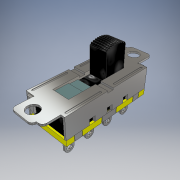
# Autodesk Inventor part: Switch-46300LDRX
Saved by Autodesk Inventor 2018 (Build 220112000, 112)
## iProperties
Created: 2021-02-17
Part Number: Switch-46300LDRX
Material: Všeobecné
Document SubType Name: Modeling
Designer: Jozko Mrkvicka
Density: 1 g/cm^3
Appearance: Výchozí
Author: Jozko Mrkvicka
Autodesk Inventor part; units mm, degrees
ref_plane "YZ Plane" through (0, 0, 0) normal (1, 0, 0) x (0, 1, 0)
ref_plane "XZ Plane" through (0, 0, 0) normal (0, 1, 0) x (-1, 0, 0)
sketch "Náčrt1" plane through (0, 0, 0) normal (0, 1, 0) x (-1, 0, 0)
  line L0 (-2.54, 20.955) -> (2.54, 20.955)
  line L1 (2.54, -20.955) -> (-2.54, -20.955)
  line L2 (-3.81, -19.685) -> (-3.81, -15.24)
  line L3 (3.81, 19.685) -> (3.81, 15.24)
  line L4 (5.715, -14.605) -> (5.715, -18.415)
  line L5 (4.445, -19.685) -> (3.81, -19.685)
  line L6 (-5.715, 14.605) -> (-5.715, 18.415)
  line L7 (-4.445, 19.685) -> (-3.81, 19.685)
  circle A0 centre (0, -17.78) radius 1.905
  circle A1 centre (0, 17.78) radius 1.905
  line L8 (-2.8575, 9.8425) -> (2.8575, 9.8425)
  line L9 (2.8575, -9.8425) -> (-2.8575, -9.8425)
  line L10 (6.985, -14.605) -> (5.715, -14.605)
  line L11 (-5.715, -14.605) -> (-6.985, -14.605)
  line L12 (6.985, 14.605) -> (6.985, 0.9525)
  line L13 (6.985, -0.9525) -> (6.985, -14.605)
  line L14 (3.81, 19.685) -> (3.81, 15.24)
  line L15 (3.81, -19.685) -> (3.81, -19.685)
  line L16 (2.8575, 9.8425) -> (2.8575, 0.9525)
  line L17 (2.8575, -0.9525) -> (2.8575, -9.8425)
  line L18 (-6.985, 0.9525) -> (-2.8575, 0.9525)
  line L19 (2.8575, 0.9525) -> (6.985, 0.9525)
  line L20 (6.985, -0.9525) -> (2.8575, -0.9525)
  line L21 (-2.8575, -0.9525) -> (-6.985, -0.9525)
  line L22 (-2.8575, -9.8425) -> (-2.8575, -0.9525)
  line L23 (-2.8575, 0.9525) -> (-2.8575, 9.8425)
  line L24 (-3.81, -20.955) -> (-3.81, -15.24)
  line L25 (-3.81, 19.685) -> (-3.81, 19.685)
  line L26 (-6.985, -14.605) -> (-6.985, -0.9525)
  line L27 (-6.985, 0.9525) -> (-6.985, 14.605)
  line L28 (6.985, 14.605) -> (5.715, 14.605)
  line L29 (-5.715, 14.605) -> (-6.985, 14.605)
  arc A2 (3.81, 19.685) -> (2.54, 20.955) centre (2.54, 19.685) ccw
  arc A3 (-2.54, 20.955) -> (-3.81, 19.685) centre (-2.54, 19.685) ccw
  arc A4 (-4.445, 19.685) -> (-5.715, 18.415) centre (-4.445, 18.415) ccw
  arc A5 (4.445, -19.685) -> (5.715, -18.415) centre (4.445, -18.415) ccw
  arc A6 (-3.81, -19.685) -> (-2.54, -20.955) centre (-2.54, -19.685) ccw
  arc A7 (2.54, -20.955) -> (3.81, -19.685) centre (2.54, -19.685) ccw
  line L30 (-5.715, -14.605) -> (-5.715, -15.24)
  line L31 (-5.715, -15.24) -> (-3.81, -15.24)
  line L32 (5.715, 14.605) -> (5.715, 15.24)
  line L33 (5.715, 15.24) -> (3.81, 15.24)
  point P0 (0, 0)
  dimension "d14" = 1.27
  dimension "d15" = 1.27
  constraints: 68 end point, 18 parallel, 12 point on circle, 12 tangent, 8 centre point, 6 horizontal, 4 equal radius, 4 perpendicular, 2 point on line, 4 other
  measures "d14" radius of A2
  measures "d15" radius of A3
extrude "Vysunutí1" add sketch "Náčrt1" along normal blind 0.635
sketch "Náčrt2" plane through (0, 0, 0) normal (0, -1, 0) x (1, 0, 0)
  line L0 (5.715, 14.605) -> (6.985, 14.605) projected
  line L1 (-6.985, -0.9525) -> (-6.985, -14.605) projected
  line L2 (6.985, 14.605) -> (-6.985, 14.605)
  line L3 (-6.985, 14.605) -> (-6.985, -14.605)
  line L4 (-6.985, -14.605) -> (6.985, -14.605)
  line L5 (6.985, -14.605) -> (6.985, 14.605)
  constraints: 8 end point, 2 parallel, 1 horizontal, 1 perpendicular
extrude "Vysunutí2" add sketch "Náčrt2" along normal blind 6.35
sketch "Náčrt3" plane through (0, 0.635, 0) normal (0, 1, 0) x (1, 0, 0)
  line L0 (-5.715, -2.54) -> (-5.715, -13.335)
  line L1 (-6.35, -13.335) -> (-6.35, -2.54)
  arc A0 (-6.35, -13.335) -> (-5.715, -13.335) centre (-6.0325, -13.335) ccw
  arc A1 (-5.715, -2.54) -> (-6.35, -2.54) centre (-6.0325, -2.54) ccw
  line L2 (-5.715, 2.54) -> (-5.715, 13.335)
  line L3 (-6.35, 13.335) -> (-6.35, 2.54)
  arc A2 (-5.715, 13.335) -> (-6.35, 13.335) centre (-6.0325, 13.335) ccw
  arc A3 (-6.35, 2.54) -> (-5.715, 2.54) centre (-6.0325, 2.54) ccw
  line L4 (5.715, -2.54) -> (5.715, -13.335)
  line L5 (6.35, -13.335) -> (6.35, -2.54)
  arc A4 (5.715, -13.335) -> (6.35, -13.335) centre (6.0325, -13.335) ccw
  arc A5 (6.35, -2.54) -> (5.715, -2.54) centre (6.0325, -2.54) ccw
  line L6 (5.715, 2.54) -> (5.715, 13.335)
  line L7 (6.35, 13.335) -> (6.35, 2.54)
  arc A6 (6.35, 13.335) -> (5.715, 13.335) centre (6.0325, 13.335) ccw
  arc A7 (5.715, 2.54) -> (6.35, 2.54) centre (6.0325, 2.54) ccw
  point P0 (-6.985, -0.9525)
  constraints: 16 end point, 16 point on circle, 8 centre point, 1 parallel
extrude "Vysunutí3" cut sketch "Náčrt3" against normal blind 0.1588
sketch "Náčrt4" plane through (0, 0, 0) normal (0, 1, 0) x (1, 0, 0)
  line L0 (2.8575, -0.9525) -> (2.8575, -9.8425) projected
  line L1 (-2.8575, -9.8425) -> (2.8575, -9.8425)
  line L2 (2.8575, -9.8425) -> (2.8575, -2.8575)
  line L3 (2.8575, -2.8575) -> (-2.8575, -2.8575)
  line L4 (-2.8575, -2.8575) -> (-2.8575, -9.8425)
  point P0 (0, 0)
  dimension "d30" = 6.985
  constraints: 8 end point, 2 parallel, 1 horizontal, 1 perpendicular, 1 point on line
  measures "d30" distance of L2.end L1.end
extrude "Vysunutí4" add sketch "Náčrt4" along normal blind 8.89
sketch "Náčrt5" plane through (2.8575, 0.635, 2.8575) normal (1, 0, 0) x (0, 0, -1)
  arc A0 (0, 7.3576) -> (-6.985, 7.3576) centre (-3.4925, 1.0099) ccw
  line L0 (0, 8.7121) -> (-6.985, 8.7121)
  line L1 (-6.985, 7.3576) -> (-6.985, 8.7121)
  line L2 (0, 7.3576) -> (0, 8.7121)
  constraints: 6 end point, 2 point on circle, 1 centre point
extrude "Vysunutí5" cut sketch "Náčrt5" against normal up to next
sketch "Náčrt6" plane through (2.8575, 0.635, 9.8425) normal (1, 0, 0) x (0, 0, -1)
  circle A0 centre (0.5108, 7.613) radius 0.3175
  circle A1 centre (1.2173, 7.8885) radius 0.3175
  circle A2 centre (1.9488, 8.0886) radius 0.3175
  circle A3 centre (2.6971, 8.2112) radius 0.3175
  circle A4 centre (3.4542, 8.2549) radius 0.3175
  circle A5 centre (4.2118, 8.2192) radius 0.3175
  circle A6 centre (4.9614, 8.1045) radius 0.3175
  circle A7 centre (5.6949, 7.9121) radius 0.3175
  circle A8 centre (6.4043, 7.6441) radius 0.3175
  point P0 (3.4925, 1.0099)
  point P1 (9.8425, -0.635)
  point P2 (3.4925, 1.0099)
  point P3 (3.4925, 1.0099)
  point P4 (3.4925, 1.0099)
  point P5 (3.4925, 1.0099)
  point P6 (3.4925, 1.0099)
  point P7 (3.4925, 1.0099)
  point P8 (3.4925, 1.0099)
  point P9 (3.4925, 1.0099)
  dimension "d38" = 48
  constraints: 9 centre point, 1 coincident, 24 other
extrude "Vysunutí6" add sketch "Náčrt6" against normal up to surface (5.715 mm away)
sketch "Náčrt7" plane through (0, 0, 0) normal (0, 1, 0) x (1, 0, 0)
  line L0 (2.8575, 0.9525) -> (2.8575, 9.8425) projected
  line L1 (-2.8575, -2.8575) -> (2.8575, -2.8575)
  line L2 (2.8575, -2.8575) -> (2.8575, 4.7625)
  line L3 (2.8575, 4.7625) -> (-2.8575, 4.7625)
  line L4 (-2.8575, 4.7625) -> (-2.8575, -2.8575)
  point P0 (0, 0)
  dimension "d42" = 7.62
  constraints: 8 end point, 2 parallel, 1 horizontal, 1 perpendicular, 1 point on line
  measures "d42" distance of L2.end L1.end
extrude "Vysunutí7" cut sketch "Náčrt7" against normal blind 0.3175
sketch "Náčrt8" plane through (0, -0.3175, 0) normal (0, 1, 0) x (1, 0, 0)
  line L0 (2.8575, -2.8575) -> (-2.8575, -2.8575) projected
  line L1 (2.8575, 4.7625) -> (2.8575, -2.8575) projected
  line L2 (-2.8575, -2.8575) -> (2.8575, -2.8575)
  line L3 (2.8575, -2.8575) -> (2.8575, 1.5875)
  line L4 (2.8575, 1.5875) -> (-2.8575, 1.5875)
  line L5 (-2.8575, 1.5875) -> (-2.8575, -2.8575)
  point P0 (0, 0)
  dimension "d45" = 4.445
  constraints: 8 end point, 2 parallel, 1 horizontal, 1 perpendicular, 1 point on line
  measures "d45" distance of L3.end L2.end
extrude "Vysunutí8" cut sketch "Náčrt8" against normal blind 0.3175
sketch "Náčrt9" plane through (0, -6.35, 0) normal (0, -1, 0) x (1, 0, 0)
  line L0 (6.35, 2.8575) -> (6.985, 2.8575)
  line L1 (6.985, -2.8575) -> (6.35, -2.8575)
  line L2 (6.35, -2.8575) -> (6.35, 2.8575)
  line L3 (-6.985, 2.8575) -> (-6.35, 2.8575)
  line L4 (-6.35, 2.8575) -> (-6.35, -2.8575)
  line L5 (-6.35, -2.8575) -> (-6.985, -2.8575)
  line L6 (6.35, 12.065) -> (6.35, 9.525)
  line L7 (6.35, 9.525) -> (6.985, 9.525)
  line L8 (6.985, 12.065) -> (6.35, 12.065)
  line L9 (-6.985, 12.065) -> (-6.35, 12.065)
  line L10 (-6.35, 12.065) -> (-6.35, 9.525)
  line L11 (-6.35, 9.525) -> (-6.985, 9.525)
  line L12 (6.985, -12.065) -> (6.35, -12.065)
  line L13 (6.35, -12.065) -> (6.35, -9.525)
  line L14 (6.35, -9.525) -> (6.985, -9.525)
  line L15 (-6.985, -12.065) -> (-6.35, -12.065)
  line L16 (-6.35, -12.065) -> (-6.35, -9.525)
  line L17 (-6.35, -9.525) -> (-6.985, -9.525)
  line L18 (6.985, 14.605) -> (-6.985, 14.605) projected
  line L19 (6.985, 14.605) -> (-6.985, 14.605)
  line L20 (-6.985, -14.605) -> (6.985, -14.605)
  line L21 (6.985, 12.065) -> (6.985, 14.605)
  line L22 (6.985, 2.8575) -> (6.985, 9.525)
  line L23 (6.985, -14.605) -> (6.985, -12.065)
  line L24 (6.985, -9.525) -> (6.985, -2.8575)
  line L25 (-6.985, -12.065) -> (-6.985, -14.605)
  line L26 (-6.985, -2.8575) -> (-6.985, -9.525)
  line L27 (-6.985, 14.605) -> (-6.985, 12.065)
  line L28 (-6.985, 9.525) -> (-6.985, 2.8575)
  point P0 (0, 0)
  point P1 (6.985, 0)
  point P2 (-6.985, 0)
  constraints: 56 end point, 22 parallel, 8 perpendicular, 6 horizontal, 3 point on line
extrude "Vysunutí9" add sketch "Náčrt9" along normal blind 1.905
sketch "Náčrt10" plane through (0, -6.35, 0) normal (0, -1, 0) x (1, 0, 0)
  line L0 (-6.985, -11.938) -> (-6.477, -11.938)
  line L1 (-6.477, -11.938) -> (-6.477, -9.652)
  line L2 (-6.477, -9.652) -> (-6.985, -9.652)
  line L3 (-6.477, 9.652) -> (-6.985, 9.652)
  line L4 (-6.985, 11.938) -> (-6.477, 11.938)
  line L5 (-6.477, 11.938) -> (-6.477, 9.652)
  line L6 (6.477, 9.652) -> (6.985, 9.652)
  line L7 (6.985, 11.938) -> (6.477, 11.938)
  line L8 (6.477, 11.938) -> (6.477, 9.652)
  line L9 (6.477, -11.938) -> (6.985, -11.938)
  line L10 (6.985, -9.652) -> (6.477, -9.652)
  line L11 (6.477, -9.652) -> (6.477, -11.938)
  line L12 (-6.477, -2.54) -> (-6.985, -2.54)
  line L13 (-6.985, 2.54) -> (-6.477, 2.54)
  line L14 (-6.477, 2.54) -> (-6.477, -2.54)
  line L15 (6.477, -2.54) -> (6.985, -2.54)
  line L16 (6.985, 2.54) -> (6.477, 2.54)
  line L17 (6.477, 2.54) -> (6.477, -2.54)
  line L18 (-6.985, -11.938) -> (-6.985, -9.652)
  line L19 (-6.985, -2.54) -> (-6.985, 2.54)
  line L20 (-6.985, 9.652) -> (-6.985, 11.938)
  line L21 (6.985, 9.652) -> (6.985, 11.938)
  line L22 (6.985, -2.54) -> (6.985, 2.54)
  line L23 (6.985, -11.938) -> (6.985, -9.652)
  point P0 (0, 0)
  point P1 (-6.985, -10.795)
  point P2 (-6.985, 10.795)
  point P3 (6.985, 10.795)
  point P4 (6.985, -10.795)
  point P5 (-6.985, 0)
  point P6 (6.985, 0)
  constraints: 48 end point, 6 horizontal, 6 parallel, 1 perpendicular
extrude "Vysunutí10" add sketch "Náčrt10" along normal blind 1.905
ref_plane "Pracovní rovina1" through (-6.477, -6.35, -2.54) normal (0, -1, 0) x (1, 0, 0)
split_face "Rozdělit1"
sketch "Náčrt11" plane through (0, -8.255, 0) normal (0, -1, 0) x (1, 0, 0)
  line L0 (-6.985, -12.065) -> (-6.985, -14.605) projected
  line L1 (-3.4925, -12.3896) -> (-3.4925, -9.2087)
  line L2 (-2.8575, -9.2087) -> (-2.8575, -12.3896)
  arc A0 (-3.4925, -9.2087) -> (-4.3905, -8.3107) centre (-4.5023, -9.3205) ccw
  arc A1 (-2.8575, -9.2087) -> (-4.0571, -7.7332) centre (-4.5023, -9.3205) ccw
  arc A2 (-2.8575, -12.3896) -> (-1.9595, -13.2876) centre (-1.8477, -12.2777) ccw
  arc A3 (-3.4925, -12.3896) -> (-2.3035, -13.8835) centre (-1.9595, -12.3896) ccw
  line L3 (-1.9595, -13.2876) -> (-2.3035, -13.8835)
  line L4 (-4.3905, -8.3107) -> (-4.0571, -7.7332)
  line L5 (-4.3905, -1.1733) -> (-4.0571, -0.5958)
  arc A4 (-2.8575, -2.0713) -> (-4.0571, -0.5958) centre (-4.5023, -2.1831) ccw
  arc A5 (-3.4925, -2.0713) -> (-4.3905, -1.1733) centre (-4.5023, -2.1831) ccw
  line L6 (-3.4925, -5.2522) -> (-3.4925, -2.0713)
  line L7 (-2.8575, -2.0713) -> (-2.8575, -5.2522)
  arc A6 (-2.8575, -5.2522) -> (-1.9595, -6.1502) centre (-1.8477, -5.1403) ccw
  arc A7 (-3.4925, -5.2522) -> (-2.3035, -6.7461) centre (-1.9595, -5.2522) ccw
  line L8 (-1.9595, -6.1502) -> (-2.3035, -6.7461)
  line L9 (-4.3905, 5.9641) -> (-4.0571, 6.5416)
  arc A8 (-2.8575, 5.0661) -> (-4.0571, 6.5416) centre (-4.5023, 4.9543) ccw
  arc A9 (-3.4925, 5.0661) -> (-4.3905, 5.9641) centre (-4.5023, 4.9543) ccw
  line L10 (-3.4925, 1.8852) -> (-3.4925, 5.0661)
  line L11 (-2.8575, 5.0661) -> (-2.8575, 1.8852)
  arc A10 (-2.8575, 1.8852) -> (-1.9595, 0.9872) centre (-1.8477, 1.9971) ccw
  arc A11 (-3.4925, 1.8852) -> (-2.3035, 0.3913) centre (-1.9595, 1.8852) ccw
  line L12 (-1.9595, 0.9872) -> (-2.3035, 0.3913)
  line L13 (-4.3905, 13.1015) -> (-4.0571, 13.679)
  arc A12 (-2.8575, 12.2035) -> (-4.0571, 13.679) centre (-4.5023, 12.0917) ccw
  arc A13 (-3.4925, 12.2035) -> (-4.3905, 13.1015) centre (-4.5023, 12.0917) ccw
  line L14 (-3.4925, 9.0226) -> (-3.4925, 12.2035)
  line L15 (-2.8575, 12.2035) -> (-2.8575, 9.0226)
  arc A14 (-2.8575, 9.0226) -> (-1.9595, 8.1246) centre (-1.8477, 9.1345) ccw
  arc A15 (-3.4925, 9.0226) -> (-2.3035, 7.5287) centre (-1.9595, 9.0226) ccw
  line L16 (-1.9595, 8.1246) -> (-2.3035, 7.5287)
  point P0 (-3.175, -10.7991)
  point P1 (-3.175, -3.6617)
  point P2 (-3.175, 3.4757)
  point P3 (-3.175, 10.6131)
  dimension "d84" = 7.1374
  constraints: 32 end point, 32 point on circle, 16 centre point, 4 concentric, 2 parallel, 1 tangent, 1 vertical, 64 other
  measures "d84" distance of L4.end L5.end
extrude "Vysunutí11" add sketch "Náčrt11" along normal blind 0.635
sketch "Náčrt12" plane through (0, -8.89, 0) normal (0, -1, 0) x (1, 0, 0)
  line L0 (-3.4925, -12.3896) -> (-3.4925, -9.2087) projected
  line L1 (-2.8575, -9.2087) -> (-2.8575, -12.3896) projected
  line L2 (-3.4925, -12.3866) -> (-2.8575, -12.3866)
  line L3 (-2.8575, -12.3866) -> (-2.8575, -9.2116)
  line L4 (-2.8575, -9.2116) -> (-3.4925, -9.2116)
  line L5 (-3.4925, -9.2116) -> (-3.4925, -12.3866)
  line L6 (-3.4925, -2.0742) -> (-3.4925, -5.2492)
  line L7 (-3.4925, -5.2492) -> (-2.8575, -5.2492)
  line L8 (-2.8575, -2.0742) -> (-3.4925, -2.0742)
  line L9 (-2.8575, -5.2492) -> (-2.8575, -2.0742)
  line L10 (-3.4925, 5.0632) -> (-3.4925, 1.8882)
  line L11 (-3.4925, 1.8882) -> (-2.8575, 1.8882)
  line L12 (-2.8575, 5.0632) -> (-3.4925, 5.0632)
  line L13 (-2.8575, 1.8882) -> (-2.8575, 5.0632)
  line L14 (-3.4925, 12.2006) -> (-3.4925, 9.0256)
  line L15 (-3.4925, 9.0256) -> (-2.8575, 9.0256)
  line L16 (-2.8575, 12.2006) -> (-3.4925, 12.2006)
  line L17 (-2.8575, 9.0256) -> (-2.8575, 12.2006)
  point P0 (0, 0)
  point P1 (-3.175, -10.7991)
  dimension "d91" = 3.175
  dimension "d94" = 7.1374
  constraints: 32 end point, 2 parallel, 1 collinear, 1 horizontal, 1 perpendicular, 1 point on line, 1 vertical, 23 other
  measures "d91" distance of L3.end L2.end
  measures "d94" distance of L4.end L6.start
extrude "Vysunutí12" add sketch "Náčrt12" along normal blind 6.35
sketch "Náčrt13" plane through (-3.4925, -8.255, -12.3896) normal (-1, 0, 0) x (0, 0, 1)
  line L0 (3.1779, -1.27) -> (3.1779, -3.81)
  line L1 (0, -3.81) -> (0, -1.27)
  line L2 (2.5415, -1.27) -> (2.5415, -3.81)
  line L3 (0.6365, -3.81) -> (0.6365, -1.27)
  arc A0 (0.0029, -5.3975) -> (3.1779, -5.3975) centre (1.5904, -5.3975) ccw
  circle A1 centre (1.5904, -5.3975) radius 0.9525
  line L4 (3.175, -1.27) -> (2.5415, -1.27)
  line L5 (0.6365, -1.27) -> (0, -1.27)
  line L6 (0, -1.27) -> (0.6365, -1.27)
  line L7 (2.5415, -1.27) -> (3.1779, -1.27)
  line L8 (3.1779, -3.81) -> (2.5415, -3.81)
  line L9 (0.6365, -3.81) -> (0, -3.81)
  line L10 (3.1779, -5.3975) -> (3.1779, -7.479)
  line L11 (3.1779, -7.479) -> (0.0029, -7.479)
  line L12 (0.0029, -7.479) -> (0.0029, -5.3975)
  circle A2 centre (8.7278, -5.3975) radius 0.9525
  arc A3 (7.1403, -5.3975) -> (10.3153, -5.3975) centre (8.7278, -5.3975) ccw
  line L13 (10.3153, -7.479) -> (7.1403, -7.479)
  line L14 (7.1403, -7.479) -> (7.1403, -5.3975)
  line L15 (10.3153, -5.3975) -> (10.3153, -7.479)
  line L16 (10.3153, -3.81) -> (9.6789, -3.81)
  line L17 (7.7739, -3.81) -> (7.1374, -3.81)
  line L18 (10.3124, -1.27) -> (9.6789, -1.27)
  line L19 (9.6789, -1.27) -> (10.3153, -1.27)
  line L20 (7.7739, -3.81) -> (7.7739, -1.27)
  line L21 (7.1374, -3.81) -> (7.1374, -1.27)
  line L22 (7.7739, -1.27) -> (7.1374, -1.27)
  line L23 (7.1374, -1.27) -> (7.7739, -1.27)
  line L24 (9.6789, -1.27) -> (9.6789, -3.81)
  line L25 (10.3153, -1.27) -> (10.3153, -3.81)
  circle A4 centre (15.8652, -5.3975) radius 0.9525
  arc A5 (14.2777, -5.3975) -> (17.4527, -5.3975) centre (15.8652, -5.3975) ccw
  line L26 (17.4527, -7.479) -> (14.2777, -7.479)
  line L27 (14.2777, -7.479) -> (14.2777, -5.3975)
  line L28 (17.4527, -5.3975) -> (17.4527, -7.479)
  line L29 (17.4527, -3.81) -> (16.8163, -3.81)
  line L30 (14.9113, -3.81) -> (14.2748, -3.81)
  line L31 (17.4498, -1.27) -> (16.8163, -1.27)
  line L32 (16.8163, -1.27) -> (17.4527, -1.27)
  line L33 (14.9113, -3.81) -> (14.9113, -1.27)
  line L34 (14.2748, -3.81) -> (14.2748, -1.27)
  line L35 (14.9113, -1.27) -> (14.2748, -1.27)
  line L36 (14.2748, -1.27) -> (14.9113, -1.27)
  line L37 (16.8163, -1.27) -> (16.8163, -3.81)
  line L38 (17.4527, -1.27) -> (17.4527, -3.81)
  circle A6 centre (23.0026, -5.3975) radius 0.9525
  arc A7 (21.4151, -5.3975) -> (24.5901, -5.3975) centre (23.0026, -5.3975) ccw
  line L39 (24.5901, -7.479) -> (21.4151, -7.479)
  line L40 (21.4151, -7.479) -> (21.4151, -5.3975)
  line L41 (24.5901, -5.3975) -> (24.5901, -7.479)
  line L42 (24.5901, -3.81) -> (23.9537, -3.81)
  line L43 (22.0487, -3.81) -> (21.4122, -3.81)
  line L44 (24.5872, -1.27) -> (23.9537, -1.27)
  line L45 (23.9537, -1.27) -> (24.5901, -1.27)
  line L46 (22.0487, -3.81) -> (22.0487, -1.27)
  line L47 (21.4122, -3.81) -> (21.4122, -1.27)
  line L48 (22.0487, -1.27) -> (21.4122, -1.27)
  line L49 (21.4122, -1.27) -> (22.0487, -1.27)
  line L50 (23.9537, -1.27) -> (23.9537, -3.81)
  line L51 (24.5901, -1.27) -> (24.5901, -3.81)
  point P0 (0, 0)
  point P1 (12.3896, 8.255)
  dimension "d109" = 7.1374
  constraints: 104 end point, 8 centre point, 8 point on circle, 7 parallel, 4 coincident, 3 horizontal, 2 perpendicular, 1 collinear, 89 other
  measures "d109" distance of L10.start L15.start
extrude "Vysunutí13" cut sketch "Náčrt13" against normal up to next
sketch "Náčrt14" plane through (6.985, -6.35, -14.605) normal (0, 0, -1) x (-1, 0, 0)
  line L0 (0, 6.985) -> (0.635, 6.985)
  line L1 (13.97, 6.985) -> (13.335, 6.985)
  line L2 (13.335, 6.35) -> (0.635, 6.35)
  line L3 (0.635, 6.35) -> (0.635, 0)
  line L4 (0.635, 0) -> (13.335, 0)
  line L5 (13.335, 0) -> (13.335, 6.35)
  point P0 (6.985, 6.35)
  constraints: 12 end point, 3 horizontal, 2 parallel, 1 perpendicular
extrude "Vysunutí14" cut sketch "Náčrt14" against normal blind 0.635
sketch "Náčrt15" plane through (-6.985, -6.35, 14.605) normal (0, 0, 1) x (1, 0, 0)
  line L0 (13.335, 6.35) -> (0.635, 6.35) projected
  line L1 (13.335, 0) -> (13.335, 6.35) projected
  line L2 (0.635, 0) -> (13.335, 0) projected
  line L3 (0.635, 6.35) -> (0.635, 0) projected
  point P0 (6.985, 6.35)
extrude "Vysunutí15" cut sketch "Náčrt15" against normal blind 0.635
sketch "Náčrt16" plane through (0, 0, 0) normal (0, -1, 0) x (1, 0, 0)
  line L0 (-5.715, 15.24) -> (-3.81, 15.24)
  line L1 (-3.81, 15.24) -> (-3.81, 14.605)
  line L2 (-3.81, 14.605) -> (-5.715, 14.605)
  line L3 (-5.715, 14.605) -> (-5.715, 15.24)
  line L4 (5.715, -15.24) -> (3.81, -15.24) projected
  line L5 (5.715, -15.24) -> (3.81, -15.24)
  line L6 (3.81, -15.24) -> (3.81, -14.605)
  line L7 (3.81, -14.605) -> (5.715, -14.605)
  line L8 (5.715, -14.605) -> (5.715, -15.24)
  point P0 (0, 0)
  dimension "d120" = 1.905
  dimension "d121" = 0.635
  constraints: 16 end point, 4 parallel, 2 horizontal, 2 perpendicular
  measures "d120" distance of L6.end L7.end
  measures "d121" distance of L5.end L6.end
extrude "Vysunutí16" add sketch "Náčrt16" along normal blind 4.445
fillet "Zaoblení1" radius 1.905 2 edges at (5.715, -4.445, -14.9225) (-5.715, -4.445, 14.9225)
fillet "Zaoblení2" radius 0.635 2 edges at (-4.7625, 0.635, 15.24) (4.7625, 0.635, -15.24)
fillet "Zaoblení3" radius 0.3175 2 edges at (-4.7625, 0, 14.605) (4.7625, 0, -14.605)
sketch "Náčrt18" plane through (6.985, 0, 0.9525) normal (1, 0, 0) x (0, 0, -1)
  line L0 (-8.5725, -6.35) -> (-1.905, -6.35) projected
  line L1 (-1.5875, -6.35) -> (3.4925, -6.35) projected
  line L2 (3.81, -6.35) -> (10.4775, -6.35) projected
  line L3 (0, -6.35) -> (0, -4.445)
  line L4 (0, -4.445) -> (1.905, -4.445)
  line L5 (1.905, -4.445) -> (1.905, -6.35)
  line L6 (6.1912, -6.35) -> (6.1912, -4.445)
  line L7 (6.1912, -4.445) -> (8.0963, -4.445)
  line L8 (8.0963, -4.445) -> (8.0963, -6.35)
  line L9 (-4.2863, -6.35) -> (-4.2863, -4.445)
  line L10 (-4.2863, -4.445) -> (-6.1913, -4.445)
  line L11 (-6.1913, -4.445) -> (-6.1913, -6.35)
  line L12 (10.6045, -6.35) -> (10.6045, -8.255) projected
  line L13 (-6.1913, -6.35) -> (-4.2863, -6.35)
  line L14 (0, -6.35) -> (1.905, -6.35)
  line L15 (6.1912, -6.35) -> (8.0963, -6.35)
  point P0 (0.9525, 0)
  point P1 (0.9525, -6.35)
  point P2 (7.1437, -6.35)
  point P3 (-5.2388, -6.35)
  constraints: 24 end point, 7 point on line, 3 midpoint, 3 parallel, 3 perpendicular
extrude "Vysunutí17" cut sketch "Náčrt18" against normal blind 0.762
sketch "Náčrt19" plane through (-6.985, 0, -0.9525) normal (-1, 0, 0) x (0, 0, 1)
  line L0 (6.1913, -6.35) -> (8.0963, -6.35) projected
  line L1 (6.1913, -4.445) -> (6.1913, -6.35) projected
  line L2 (8.0963, -4.445) -> (6.1913, -4.445) projected
  line L3 (8.0963, -6.35) -> (8.0963, -4.445) projected
  line L4 (-6.1912, -4.445) -> (-6.1912, -6.35) projected
  line L5 (-4.2862, -4.445) -> (-6.1912, -4.445) projected
  line L6 (-4.2862, -6.35) -> (-4.2862, -4.445) projected
  line L7 (-6.1912, -6.35) -> (-4.2862, -6.35) projected
  line L8 (1.905, -6.35) -> (1.905, -4.445) projected
  line L9 (0, -6.35) -> (1.905, -6.35) projected
  line L10 (0, -4.445) -> (0, -6.35) projected
  line L11 (1.905, -4.445) -> (0, -4.445) projected
  point P0 (0.9525, 0)
extrude "Vysunutí18" cut sketch "Náčrt19" against normal blind 0.762
